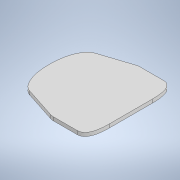
# Autodesk Inventor part: Base del Robot
Saved by Autodesk Inventor 2022.2 (Build 262287010, 287A)
## iProperties
Created: 2022-03-28
Part Number: Base del Robot
Material: Generic
Document SubType Name: Modeling
Designer: Santiago Larraín
Density: 1 g/cm^3
Appearance: Default
Author: Santiago Larraín
Autodesk Inventor part; units mm, degrees
ref_plane "YZ Plane" through (0, 0, 0) normal (1, 0, 0) x (0, 1, 0)
ref_plane "XZ Plane" through (0, 0, 0) normal (0, 1, 0) x (-1, 0, 0)
ref_plane "XY Plane" through (0, 0, 0) normal (0, 0, 1) x (1, 0, 0)
sketch "Sketch1" plane through (0, 0, 0) normal (0, 1, 0) x (-1, 0, 0)
  line L0 (-92.5, 115) -> (92.5, -115) construction
  line L1 (-92.5, -115) -> (92.5, 115) construction
  line L2 (-75.8, 45) -> (-75.8, -45)
  line L3 (-75.8, 91.5) -> (75.8, -91.5) construction
  line L4 (-75.8, -91.5) -> (75.8, 91.5) construction
  line L5 (-75.8, 0) -> (-75.8, -45)
  line L6 (-75.8, -45) -> (-75.8, -91.5) construction
  line L7 (-75.8, -91.5) -> (-53.7188, -91.5) construction
  spline S0 degree 2 poles (-75.8, -45) (-75.8, -91.5) (-53.7188, -91.5) knots 1 1 1 2 2 2
  line L8 (-75.8, 0) -> (-75.8, 45)
  line L9 (-75.8, 45) -> (-75.8, 91.5) construction
  line L10 (-75.8, 91.5) -> (-53.7188, 91.5) construction
  spline S1 degree 2 poles (-75.8, 45) (-75.8, 91.5) (-53.7188, 91.5) knots 1 1 1 2 2 2
  line L11 (-73.5978, 91.5) -> (-75.8, 91.5)
  line L12 (-75.8, -91.5) -> (-73.5978, -91.5)
  line L13 (0, 91.5) -> (75.8, 66.8711)
  line L14 (0, 91.5) -> (79.7008, 91.5) construction
  line L15 (0, -91.5) -> (75.8, -66.8711)
  line L16 (73.5978, -91.5) -> (79.7008, -91.5) construction
  line L17 (96.8, 0) -> (96.8, 45) construction
  line L18 (96.8, 45) -> (75.8, 66.8711) construction
  spline S2 degree 2 poles (96.8, 0) (96.8, 45) (75.8, 66.8711) knots 1 1 1 2 2 2
  line L19 (96.8, 0) -> (96.8, -45) construction
  line L20 (96.8, -45) -> (75.8, -66.8711) construction
  spline S3 degree 2 poles (96.8, 0) (96.8, -45) (75.8, -66.8711) knots 1 1 1 2 2 2
  line L21 (75.8, 91.5) -> (73.5978, 91.5)
  line L22 (0, 91.5) -> (-53.7188, 91.5)
  line L23 (-53.7188, -91.5) -> (0, -91.5)
  line L24 (73.5978, -91.5) -> (75.8, -91.5)
  point P0 (0, 0)
  dimension "d3" = 183
  dimension "d6" = 45
  dimension "d7" = 45
  dimension "d8" = 18
  dimension "d9" = 18
  constraints: 34 end point, 9 parallel, 5 midpoint, 4 point on line, 3 perpendicular, 2 coincident, 2 collinear, 2 horizontal, 1 equal length, 1 vertical, 12 other
  measures "d3" distance of L3.start L4.start
  measures "d6" distance of L2.end L5.start
  measures "d7" distance of L2.start L5.start
  measures "d8" angle of L13 L14
  measures "d9" angle of L16 L15
extrude "Extrusion1" add sketch "Sketch1" along normal blind 7.5
fillet "Fillet1" radius 25 4 edges at (0, 3.75, 91.5) (-75.8, 3.75, 66.8711) (-75.8, 3.75, -66.8711) (0, 3.75, -91.5)
body "Solid1"
